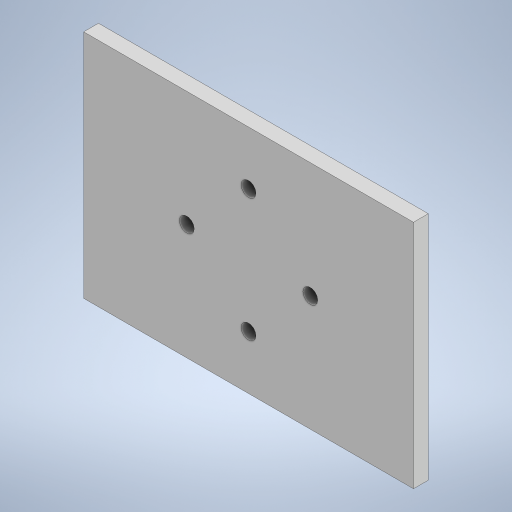
# Autodesk Inventor part: motor mount
Saved by Autodesk Inventor 2024 (Build 280153000, 153)
## iProperties
Created: 2023-07-17
Part Number: motor mount
Material: Generic
Document SubType Name: Modeling
Designer: USER
Density: 1 g/cm^3
Appearance: Default
Author: USER
Autodesk Inventor part; units mm, degrees
ref_plane "YZ Plane" through (0, 0, 0) normal (1, 0, 0) x (0, 1, 0)
ref_plane "XZ Plane" through (0, 0, 0) normal (0, 1, 0) x (-1, 0, 0)
ref_plane "XY Plane" through (0, 0, 0) normal (0, 0, 1) x (1, 0, 0)
sketch "Sketch1" plane through (0, 0, 0) normal (0, 0, 1) x (1, 0, 0)
  line L0 (33.3835, 23.3615) -> (-33.3835, 23.3615)
  line L1 (-33.3835, 23.3615) -> (-33.3835, -23.3615)
  line L2 (-33.3835, -23.3615) -> (33.3835, -23.3615)
  line L3 (33.3835, -23.3615) -> (33.3835, 23.3615)
  point P0 (0, 0)
  constraints: 8 end point, 2 parallel, 1 horizontal, 1 perpendicular
extrude "Extrusion1" add sketch "Sketch1" along normal blind 3
sketch "Sketch2" plane through (0, 0, 3) normal (0, 0, 1) x (1, 0, 0)
  circle A0 centre (-12.5, 0) radius 1.5
  circle A1 centre (0, -12.5) radius 1.5
  circle A2 centre (12.5, 0) radius 1.5
  circle A3 centre (0, 12.5) radius 1.5
  point P0 (0, 0)
  constraints: 4 centre point
extrude "Extrusion2" cut sketch "Sketch2" against normal blind 3
body "Solid1"
